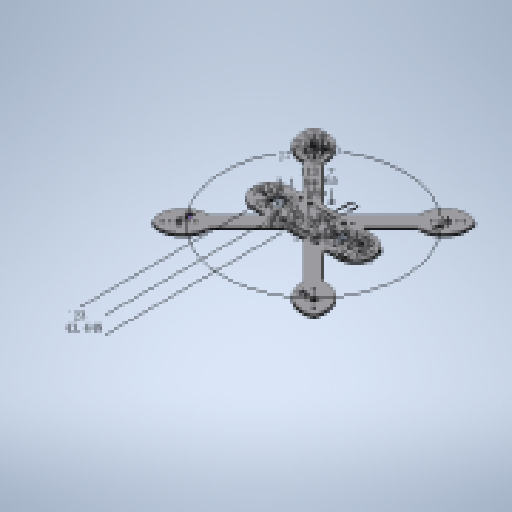
# Autodesk Inventor part: drone.bottom.plate.revision2
Saved by Autodesk Inventor 2025.2 (Build 292293000, 293)
## iProperties
Created: 2016-03-03
Part Number: drone.bottom.plate.revision2
Material: 一般
Document SubType Name: Modeling
Designer: 200288284
Density: 1 g/cm^3
Appearance: 默认值
Author: 200288284
Autodesk Inventor part; units mm, degrees
ref_plane "YZ Plane" through (0, 0, 0) normal (1, 0, 0) x (0, 1, 0)
ref_plane "XZ Plane" through (0, 0, 0) normal (0, 1, 0) x (-1, 0, 0)
ref_plane "XY Plane" through (0, 0, 0) normal (0, 0, 1) x (1, 0, 0)
ref_plane "Work Plane4" through (0, 3, 0) normal (0, 1, 0) x (1, 0, 0)
sketch "草图10" plane through (0, 3, 0) normal (0, 1, 0) x (1, 0, 0)
  line L0 (-10.6863, 22) -> (-56.6482, 67.9619)
  arc A0 (-56.6482, 67.9619) -> (-96.1665, 96.1665) centre (-84.6531, 70.5109) ccw
  arc A1 (-96.1665, 96.1665) -> (-67.9619, 56.6482) centre (-70.5109, 84.6531) ccw
  line L1 (-67.9619, 56.6482) -> (-32.3137, 21)
  line L2 (-32.3137, 21) -> (-50.3137, 21)
  arc A2 (-50.3137, 21) -> (-71.3137, 0) centre (-50.3137, 0) ccw
  circle A3 centre (-79.9031, 79.9031) radius 3.5
  arc A4 (54, 5.5) -> (54, 7.5) centre (54, 6.5) ccw
  line L3 (54, 5.5) -> (46, 5.5)
  arc A5 (46, 7.5) -> (46, 5.5) centre (46, 6.5) ccw
  line L4 (46, 7.5) -> (54, 7.5)
  line L5 (45.9, 13) -> (45.9, 15.1)
  line L6 (45.9, 15.1) -> (51.1, 15.1)
  line L7 (51.1, 15.1) -> (51.1, 13)
  line L8 (51.1, 13) -> (45.9, 13)
  line L9 (41.1, 15.1) -> (41.1, 13)
  line L10 (41.1, 13) -> (35.9, 13)
  line L11 (35.9, 13) -> (35.9, 15.1)
  line L12 (35.9, 15.1) -> (41.1, 15.1)
  circle A6 centre (51, 0) radius 1.55
  circle A7 centre (57, 15) radius 1.55
  circle A8 centre (-53.4488, 15) radius 1.55
  circle A9 centre (-30.4488, 15) radius 1.55
  line L13 (58.5, 4) -> (58.5, 9)
  line L14 (58.5, 9) -> (60.5, 9)
  line L15 (60.5, 9) -> (60.5, 4)
  line L16 (60.5, 4) -> (58.5, 4)
  line L17 (10, 10) -> (10, -10)
  line L18 (-10, -10) -> (-10, 10)
  line L19 (-10, 10) -> (10, 10)
  line L20 (-10, 0) -> (10, 0)
  line L21 (-71.3137, 0) -> (71.3137, 0)
  line L22 (0, 45) -> (0, 0)
  line L23 (-79.9031, 79.9031) -> (0, 0)
  arc A10 (-96.1665, -96.1665) -> (-56.6482, -67.9619) centre (-84.6531, -70.5109) ccw
  arc A11 (-67.9619, -56.6482) -> (-96.1665, -96.1665) centre (-70.5109, -84.6531) ccw
  arc A12 (-71.3137, 0) -> (-50.3137, -21) centre (-50.3137, 0) ccw
  line L24 (-32.3137, -21) -> (-50.3137, -21)
  line L25 (-67.9619, -56.6482) -> (-32.3137, -21)
  line L26 (-10.6863, -22) -> (-56.6482, -67.9619)
  arc A13 (96.1665, 96.1665) -> (56.6482, 67.9619) centre (84.6531, 70.5109) ccw
  arc A14 (67.9619, 56.6482) -> (96.1665, 96.1665) centre (70.5109, 84.6531) ccw
  arc A15 (71.3137, 0) -> (50.3137, 21) centre (50.3137, 0) ccw
  line L27 (32.3137, 21) -> (50.3137, 21)
  line L28 (67.9619, 56.6482) -> (32.3137, 21)
  line L29 (10.6863, 22) -> (56.6482, 67.9619)
  line L30 (10.6863, -22) -> (56.6482, -67.9619)
  arc A16 (56.6482, -67.9619) -> (96.1665, -96.1665) centre (84.6531, -70.5109) ccw
  arc A17 (96.1665, -96.1665) -> (67.9619, -56.6482) centre (70.5109, -84.6531) ccw
  line L31 (67.9619, -56.6482) -> (32.3137, -21)
  line L32 (32.3137, -21) -> (50.3137, -21)
  arc A18 (50.3137, -21) -> (71.3137, 0) centre (50.3137, 0) ccw
  line L33 (-10, -10) -> (10, -10)
  line L34 (10, 0) -> (51, 0)
  line L35 (0, 18.9948) -> (0, 0)
  line L36 (46, 6.5) -> (46, 0)
  line L37 (54, 7.5) -> (54, 5.5)
  line L38 (46, 7.5) -> (46, 5.5)
  line L39 (-10.6863, 22) -> (10.6863, 22)
  line L40 (-10.6863, -22) -> (10.6863, -22)
  line L41 (-10.6863, 22) -> (-10.6863, 0)
  circle A19 centre (-30.4488, -15) radius 1.55
  circle A20 centre (-53.4488, -15) radius 1.55
  line L42 (51.1, -15.1) -> (51.1, -13)
  line L43 (46, -7.5) -> (54, -7.5)
  arc A21 (46, -5.5) -> (46, -7.5) centre (46, -6.5) ccw
  line L44 (51.1, -13) -> (45.9, -13)
  line L45 (45.9, -15.1) -> (51.1, -15.1)
  line L46 (45.9, -13) -> (45.9, -15.1)
  line L47 (41.1, -15.1) -> (41.1, -13)
  line L48 (41.1, -13) -> (35.9, -13)
  line L49 (35.9, -15.1) -> (41.1, -15.1)
  line L50 (35.9, -13) -> (35.9, -15.1)
  line L51 (54, -5.5) -> (46, -5.5)
  arc A22 (54, -7.5) -> (54, -5.5) centre (54, -6.5) ccw
  circle A23 centre (57, -15) radius 1.55
  line L52 (58.5, -4) -> (58.5, -9)
  line L53 (58.5, -9) -> (60.5, -9)
  line L54 (60.5, -9) -> (60.5, -4)
  line L55 (60.5, -4) -> (58.5, -4)
  line L56 (54, -7.5) -> (54, -5.5)
  line L57 (46, -7.5) -> (46, -5.5)
  circle A24 centre (-79.9031, -79.9031) radius 3.5
  circle A25 centre (79.9031, 79.9031) radius 3.5
  circle A26 centre (79.9031, -79.9031) radius 3.5
  circle A27 centre (-74.2462, 74.2462) radius 1.05
  circle A28 centre (-85.5599, 85.5599) radius 1.05
  circle A29 centre (-84.1457, 75.6604) radius 1.05
  circle A30 centre (-75.6604, 84.1457) radius 1.05
  circle A31 centre (-74.2462, -74.2462) radius 1.05
  circle A32 centre (-85.5599, -85.5599) radius 1.05
  circle A33 centre (-84.1457, -75.6604) radius 1.05
  circle A34 centre (-75.6604, -84.1457) radius 1.05
  circle A35 centre (74.2462, 74.2462) radius 1.05
  circle A36 centre (85.5599, 85.5599) radius 1.05
  circle A37 centre (84.1457, 75.6604) radius 1.05
  circle A38 centre (75.6604, 84.1457) radius 1.05
  circle A39 centre (75.6604, -84.1457) radius 1.05
  circle A40 centre (74.2462, -74.2462) radius 1.05
  circle A41 centre (84.1457, -75.6604) radius 1.05
  circle A42 centre (85.5599, -85.5599) radius 1.05
  line L58 (-85.5599, 85.5599) -> (-79.9031, 79.9031)
  line L59 (-75.6604, 84.1457) -> (-84.1457, 75.6604)
  line L60 (-96.1665, 96.1665) -> (-79.9031, 79.9031)
  line L61 (-56.6482, 67.9619) -> (-67.9619, 56.6482)
  circle A43 centre (-25, -21) radius 1.55
  line L62 (-53.4488, 15) -> (-53.4488, -15)
  line L63 (-53.4488, -15) -> (-30.4488, -15)
  line L64 (-30.4488, -15) -> (-30.4488, 15)
  line L65 (-30.4488, 15) -> (-53.4488, 15)
  line L66 (57, 15) -> (57, -15)
  line L67 (-49.4488, -7.56) -> (-34.4488, -7.56)
  line L68 (-34.4488, -7.56) -> (-34.4488, 7.44)
  line L69 (-34.4488, 7.44) -> (-49.4488, 7.44)
  line L70 (-49.4488, 7.44) -> (-49.4488, -7.56)
  arc A44 (-13, -15) -> (-13, -17) centre (-13, -16) ccw
  line L71 (-13, -15) -> (12, -15)
  line L72 (12, -15) -> (-13, -15)
  line L73 (12, -17) -> (-13, -17)
  arc A45 (12, -17) -> (12, -15) centre (12, -16) ccw
  line L74 (-62.377, 0) -> (-55.4488, -4)
  line L75 (-55.4488, -4) -> (-55.4488, 4)
  line L76 (-62.377, 0) -> (-55.4488, 4)
  arc A46 (-13, 17) -> (-13, 15) centre (-13, 16) ccw
  line L77 (12, 15) -> (-13, 15)
  line L78 (12, 17) -> (-13, 17)
  arc A47 (12, 15) -> (12, 17) centre (12, 16) ccw
  line L79 (27, -7.5) -> (37, -7.5)
  line L80 (37, -7.5) -> (37, 7.5)
  line L81 (37, 7.5) -> (27, 7.5)
  line L82 (27, 7.5) -> (27, -7.5)
  line L83 (-20.0149, -19.6211) -> (-16.4087, -16.0149)
  line L84 (-16.4087, -16.0149) -> (-20.0149, -12.4087)
  line L85 (-20.0149, -12.4087) -> (-23.6211, -16.0149)
  line L86 (-23.6211, -16.0149) -> (-20.0149, -19.6211)
  line L87 (-18.2118, -14.2118) -> (-21.818, -17.818)
  line L88 (-25, -21) -> (-21.818, -17.818)
  circle A48 centre (25, -21) radius 1.55
  line L89 (20.0149, -19.6211) -> (16.4087, -16.0149)
  line L90 (16.4087, -16.0149) -> (20.0149, -12.4087)
  line L91 (20.0149, -12.4087) -> (23.6211, -16.0149)
  line L92 (23.6211, -16.0149) -> (20.0149, -19.6211)
  circle A49 centre (-25, 21) radius 1.55
  line L93 (-20.0149, 19.6211) -> (-16.4087, 16.0149)
  line L94 (-16.4087, 16.0149) -> (-20.0149, 12.4087)
  line L95 (-20.0149, 12.4087) -> (-23.6211, 16.0149)
  line L96 (-23.6211, 16.0149) -> (-20.0149, 19.6211)
  line L97 (20.0149, 19.6211) -> (16.4087, 16.0149)
  line L98 (23.6211, 16.0149) -> (20.0149, 19.6211)
  line L99 (20.0149, 12.4087) -> (23.6211, 16.0149)
  line L100 (16.4087, 16.0149) -> (20.0149, 12.4087)
  circle A50 centre (25, 21) radius 1.55
  circle A51 centre (-89.8026, 89.8026) radius 1.55
  circle A52 centre (-70.0036, 70.0036) radius 1.55
  circle A53 centre (-89.8026, -89.8026) radius 1.55
  circle A54 centre (-70.0036, -70.0036) radius 1.55
  circle A55 centre (89.8026, 89.8026) radius 1.55
  circle A56 centre (70.0036, 70.0036) radius 1.55
  circle A57 centre (89.8026, -89.8026) radius 1.55
  circle A58 centre (70.0036, -70.0036) radius 1.55
  line L101 (-69.7637, 82.6311) -> (-74.2364, 81.8751)
  arc A59 (-74.2364, 81.8751) -> (-74.2364, 77.931) centre (-73.9031, 79.9031) ccw
  line L102 (-74.2364, 77.931) -> (-69.7637, 77.175)
  line L103 (-69.7637, 77.175) -> (-56.893, 74.9995)
  line L104 (-69.7637, 82.6311) -> (-60.1232, 84.2607)
  circle A60 centre (-79.9031, 79.9031) radius 6.75
  line L105 (-73.4876, 82.0017) -> (-73.4876, 77.8045)
  circle A61 centre (-79.9031, 79.9031) radius 16.4697
  line L106 (-77.931, -74.2364) -> (-77.175, -69.7637)
  line L107 (-77.175, -69.7637) -> (-74.9995, -56.893)
  line L108 (-82.6311, -69.7637) -> (-84.2607, -60.1232)
  line L109 (-82.6311, -69.7637) -> (-81.8751, -74.2364)
  line L110 (-82.0017, -73.4876) -> (-77.8045, -73.4876)
  circle A62 centre (-79.9031, -79.9031) radius 16.4697
  line L111 (74.2364, -77.931) -> (69.7637, -77.175)
  line L112 (69.7637, -77.175) -> (56.893, -74.9995)
  line L113 (69.7637, -82.6311) -> (60.1232, -84.2607)
  line L114 (69.7637, -82.6311) -> (74.2364, -81.8751)
  line L115 (73.4876, -82.0017) -> (73.4876, -77.8045)
  circle A63 centre (79.9031, -79.9031) radius 16.4697
  line L116 (77.931, 74.2364) -> (77.175, 69.7637)
  line L117 (77.175, 69.7637) -> (74.9995, 56.893)
  line L118 (82.6311, 69.7637) -> (84.2607, 60.1232)
  line L119 (82.6311, 69.7637) -> (81.8751, 74.2364)
  line L120 (82.0017, 73.4876) -> (77.8045, 73.4876)
  circle A64 centre (79.9031, 79.9031) radius 16.4697
  point P0 (-79.9031, 79.9031)
  point P1 (49.45, 0)
  point P2 (52.55, 0)
  point P3 (-23.4486, 23.4486)
  point P4 (-22.5514, 22.5514)
  point P5 (-15.7118, 15.7118)
  point P6 (-19.318, 19.318)
  point P7 (-13.6863, 16.7373)
  point P8 (-13.6863, 17.2925)
  point P9 (-75.9031, 79.9031)
  point P10 (-64.4706, 83.5258)
  point P11 (-83.5258, -64.4706)
  point P12 (64.4706, -83.5258)
  point P13 (83.5258, 64.4706)
  point P14 (76.1772, 63.8604)
  point P15 (83.629, 63.8604)
  point P16 (63.8604, -76.1772)
  point P17 (63.8604, -83.629)
  point P18 (-76.1772, -63.8604)
  point P19 (-83.629, -63.8604)
  point P20 (-63.8604, 76.1772)
  point P21 (-63.8604, 83.629)
  dimension "d279" = 45
  dimension "d280" = 18
  dimension "d301" = 8
  dimension "d302" = 8
  dimension "d305" = 45
  dimension "d310" = 7
  dimension "d319" = 3.1
  dimension "d325" = 5
  dimension "d326" = 2
  dimension "d327" = 5.2
  dimension "d328" = 2.1
  dimension "d329" = 5.2
  dimension "d330" = 2.1
  dimension "d341" = 20
  dimension "d347" = 8
  dimension "d348" = 6.5
  dimension "d349" = 36
  dimension "d351" = 2
  dimension "d353" = 48.5
  dimension "d354" = 4
  dimension "d357" = 13
  dimension "d358" = 13
  dimension "d359" = 4.8
  dimension "d360" = 22
  dimension "d361" = 25.9
  dimension "d363" = 23
  dimension "d364" = 43.4488
  dimension "d372" = 2.1
  dimension "d373" = 2.1
  dimension "d374" = 16
  dimension "d375" = 8
  dimension "d376" = 2.1
  dimension "d377" = 2.1
  dimension "d378" = 12
  dimension "d379" = 6
  dimension "d382" = 113
  dimension "d391" = 65
  dimension "d394" = 20
  dimension "d395" = 41
  dimension "d402" = 30
  dimension "d403" = 30
  dimension "d404" = 47
  dimension "d406" = 90
  dimension "d407" = 21
  dimension "d408" = 2
  dimension "d409" = 25
  dimension "d410" = 5
  dimension "d412" = 1
  dimension "d413" = 1
  dimension "d414" = 3
  dimension "d415" = 15
  dimension "d416" = 15
  dimension "d417" = 7.56
  dimension "d418" = 4
  dimension "d421" = 8
  dimension "d422" = 6
  dimension "d427" = 10
  dimension "d428" = 15
  dimension "d429" = 7.5
  dimension "d431" = 23
  dimension "d432" = 10
  dimension "d433" = 10
  dimension "d434" = 3.1
  dimension "d437" = 17
  constraints: 246 end point, 89 symmetric about line, 65 centre point, 49 point on circle, 21 perpendicular, 19 point on line, 11 midpoint, 10 parallel, 9 equal length, 7 horizontal, 4 vertical, 3 coincident, 3 collinear, 3 equal radius, 115 other
  measures "d279" angle of L22 L23
  measures "d280" distance of L2.start L2.end
  measures "d301" distance between parallel lines of L23 L1
  measures "d302" distance between parallel lines of L0 L23
  measures "d305" distance of L22.start L22.end
  measures "d310" diameter of A3
  measures "d319" diameter of A8
  measures "d325" distance of L13.start L13.end
  measures "d326" distance of L13.end L14.end
  measures "d327" distance of L7.end L8.end
  measures "d328" distance of L8.end L6.start
  measures "d329" distance of L9.end L10.end
  measures "d330" distance of L10.end L12.start
  measures "d341" distance of L18.start L19.start
  measures "d347" distance of L4.start L4.end
  measures "d348" distance of L36.start L36.end
  measures "d349" distance between parallel lines of L17 L36
  measures "d351" distance of L4.end L37.end
  measures "d353" distance between parallel lines of L17 L13
  measures "d354" distance between parallel lines of L20 L16
  measures "d357" distance between parallel lines of L34 L10
  measures "d358" distance between parallel lines of L34 L8
  measures "d359" distance between parallel lines of L5 L9
  measures "d360" distance of L0.start L41.end
  measures "d361" distance between parallel lines of L17 L11
  measures "d363" distance of L62.start L64.end
  measures "d364" distance from line of L18 L62.start
  measures "d372" diameter of A27
  measures "d373" diameter of A28
  measures "d374" distance of A27.centre A28.centre
  measures "d375" distance of L23.start A28.centre
  measures "d376" diameter of A30
  measures "d377" diameter of A29
  measures "d378" distance of L59.start L59.end
  measures "d379" distance of L23.start L59.start
  measures "d382" distance of L23.start L22.end
  measures "d391" distance of L0.start L0.end
  measures "d394" distance between parallel lines of L17 L18
  measures "d395" distance from line of L17 L34.end
  measures "d402" distance of L62.start L62.end
  measures "d403" distance of L66.start L66.end
  measures "d404" distance from line of L17 L66.end
  measures "d407" radius of A2
  measures "d408" distance between parallel lines of L71 L73
  measures "d409" distance of L73.start L73.end
  measures "d410" distance between parallel lines of L71 L33
  measures "d412" radius of A44
  measures "d413" radius of A45
  measures "d414" distance from line of L18 A44.centre
  measures "d415" distance between parallel lines of L68 L70
  measures "d416" distance between parallel lines of L69 L67
  measures "d417" distance between parallel lines of L21 L67
  measures "d418" distance between parallel lines of L64 L68
  measures "d421" distance of L75.start L76.end
  measures "d422" distance between parallel lines of L70 L75
  measures "d427" distance between parallel lines of L80 L82
  measures "d428" distance between parallel lines of L81 L79
  measures "d429" distance between parallel lines of L79 L21
  measures "d431" distance of L60.start L23.start
  measures "d432" distance from line of L23 A1.centre
  measures "d433" distance from line of L23 A0.centre
  measures "d434" diameter of A43
  measures "d437" distance between parallel lines of L17 L82
extrude "拉伸10" add sketch "草图10" along normal blind 3 contours L41 L78 A46 L77 L23 L61 L0 | L39 L22 L78 L41 | L61 L23 A61 L103 A0 | L39 L29 A13 A14 L118 A64 L117 L28 L27 A15 L21 A6 L80 L81 L82 L17 L19 L22 L77 A47 L78 | L78 L22 L77 L41 | L41 L77 A46 L78 | L103 A61 L104 A0 | L61 A1 L60 A61 L23 | L23 L41 L21 L64 A9 L65 A8 L62 L75 L76 A2 L2 L1 L61 | L77 L22 L19 L23 L41 | L78 A47 L77 L22 | L104 A61 L60 A0 | A61 L23 A52 A27 A60 L102 L103 | L103 L102 A60 L101 L104 A61 | A61 L60 A51 A28 L58 A60 A29 L23 A27 A52 | L23 L18 L21 L41 | L104 L101 A60 A30 L58 A28 L60 A51 A61 | A52 L23 | L23 A52 | L23 L20 L18 | L19 L22 L23 | L21 L18 L33 L17 L82 L79 L80 A6 A18 L32 L31 A17 A16 L113 A63 L112 L30 L40 L26 A10 A11 L108 A62 L107 L25 L24 A12 L74 L75 L62 A20 L63 A19 L64 | L19 L17 L20 L22 | A60 L23 A3 L59 A30 L101 A59 L102 | L105 A60 | L102 A59 L101 L105 | A51 L60 | L60 A51 | L20 L17 L33 L18 | L64 A19 L63 A20 L62 L21 L70 L67 L68 | L21 L68 L69 L70 L62 A8 L65 A9 L64 | A14 L117 A64 L118 | A60 A29 L59 A3 L23 | A27 L23 | L23 A27 | L68 L67 L70 L21 | L21 L70 L69 L68 | L64 L63 A19 | A19 L63 L64 | L64 L65 A9 | A9 L65 L64 | A64 L117 L116 L120 L119 L118 | L118 L119 L120 L116 L117 A64 | A60 A30 | A30 A60 | L23 L59 A3 | A3 L59 L23 | A60 A29 | A29 A60 | L60 L58 A28 | A28 L58 L60 | L82 L81 L80 L21 | L21 L80 L79 L82 | L76 L75 L21 | L21 L75 L74 | L59 A3 L58 A60 A30 | L59 A29 A60 L58 A3 | A3 L58 L59 | L58 A3 L59 | L63 L62 A20 | A20 L62 L63 | L65 L62 A8 | A8 L62 L65 | L21 A6 | A6 L21 | L107 A62 L108 A11 | A62 L108 L109 L110 L106 L107 | L107 L106 L110 L109 L108 A62 | A16 L112 A63 L113 | A63 L112 L111 L115 L114 L113 | L113 L114 L115 L111 L112 A63 | L37 A4 | L3 L36 L38 L4 L37 | A5 L38 L36 | L5 L6 L7 L8 | L9 L10 L11 L12 | A7 | L13 L14 L15 L16 | L45 L46 L44 L42 | L57 L51 L56 L43 | A21 L57 | L56 A22 | L49 L50 L48 L47 | A23 | L55 L54 L53 L52 | A24 | A25 | A26 | A31 | A32 | A33 | A34 | A35 | A36 | A37 | A38 | A39 | A40 | A41 | A42 | A43 | L71 A45 L73 A44 | L86 L87 L84 L83 | L86 L85 L84 L87 | A48 | L89 L90 L91 L92 | A49 | L93 L94 L95 L96 | L98 L99 L100 L97 | A50 | A53 | A54 | A55 | A56 | A57 | A58
extrude "拉伸11" cut sketch "草图10" along normal blind 5 contours L64 L63 A19 | A19 L63 L64 | L64 L65 A9 | A9 L65 L64 | L63 L62 A20 | A20 L62 L63 | L65 L62 A8 | A8 L62 L65 | L5 L6 L7 L8 | L9 L10 L11 L12 | A7 | L45 L46 L44 L42 | L49 L50 L48 L47 | A23 | A43 | L86 L87 L84 L83 | L86 L85 L84 L87 | A48 | L89 L90 L91 L92 | A49 | L93 L94 L95 L96 | L98 L99 L100 L97 | A50
extrude "拉伸12" cut sketch "草图10" along normal blind 16 contours L103 L102 A60 L101 L104 A61 | A52 L23 | L23 A52 | L105 A60 | A51 L60 | L60 A51 | A27 L23 | L23 A27 | A64 L117 L116 L120 L119 L118 | A60 A30 | A30 A60 | L23 L59 A3 | A3 L59 L23 | A60 A29 | A29 A60 | L60 L58 A28 | A28 L58 L60 | A3 L58 L59 | L58 A3 L59 | L107 L106 L110 L109 L108 A62 | A63 L112 L111 L115 L114 L113 | A24 | A25 | A26 | A31 | A32 | A33 | A34 | A35 | A36 | A37 | A38 | A39 | A40 | A41 | A42 | A53 | A54 | A55 | A56 | A57 | A58 picked at (79.4859, 67.6695) picked at (-79.4859, -67.6695) picked at (67.6695, -79.4859)
extrude "拉伸14" cut sketch "草图10" along normal blind 41 contours L78 L22 L77 L41 | L41 L77 A46 L78 | L78 A47 L77 L22 | L68 L67 L70 L21 | L21 L70 L69 L68 | L82 L81 L80 L21 | L21 L80 L79 L82 | L76 L75 L21 | L21 L75 L74 | A6 L21 | L37 A4 | L3 L36 L38 L4 L37 | A5 L38 L36 | L13 L14 L15 L16 | L57 L51 L56 L43 | A21 L57 | L56 A22 | L55 L54 L53 L52 | L71 A45 L73 A44 picked at (50.5233, 0.9083)
fillet "圆角24" radius 2 1 edges at (-32.3137, 4.5, -21)
fillet "圆角25" radius 3 3 edges at (32.3137, 4.5, -21) (32.3137, 4.5, 21) (-32.3137, 4.5, 21)
fillet "圆角26" radius 10 7 edges at (-56.6482, 4.5, 67.9619) (-67.9619, 4.5, 56.6482) (56.6482, 4.5, 67.9619) (67.9619, 4.5, 56.6482) (67.9619, 4.5, -56.6482) (56.6482, 4.5, -67.9619) (-56.6482, 4.5, -67.9619)
fillet "圆角27" radius 10 4 edges at (-10.6863, 4.5, -22) (10.6863, 4.5, -22) (10.6863, 4.5, 22) (-10.6863, 4.5, 22)
fillet "圆角28" radius 5 4 edges at (96.1665, 4.5, 96.1665) (-96.1665, 4.5, 96.1665) (-96.1665, 4.5, -96.1665) (96.1665, 4.5, -96.1665)
fillet "圆角29" radius 0.5 16 edges at (-73.4876, 4.5, -82.0017) (-73.4876, 4.5, -77.8045) (-63.8604, 4.5, -83.629) (-63.8604, 4.5, -76.1772) (-83.629, 4.5, 63.8604) (-76.1772, 4.5, 63.8604) (-82.0017, 4.5, 73.4876) (-77.8045, 4.5, 73.4876) (63.8604, 4.5, 76.1772) (63.8604, 4.5, 83.629) (73.4876, 4.5, 77.8045) (73.4876, 4.5, 82.0017) (77.8045, 4.5, -73.4876) (82.0017, 4.5, -73.4876) (76.1772, 4.5, -63.8604) (83.629, 4.5, -63.8604)
